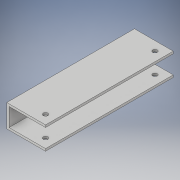
# Autodesk Inventor part: U holder
Saved by Autodesk Inventor 2017 (Build 210142000, 142)
## iProperties
Created: 2019-02-04
Part Number: U holder
Material: Generic
Document SubType Name: Modeling
Designer: S346553810
Density: 1 g/cm^3
Appearance: Default
Author: S346553810
Autodesk Inventor part; units mm, degrees
ref_plane "YZ Plane" through (0, 0, 0) normal (1, 0, 0) x (0, 1, 0)
ref_plane "XZ Plane" through (0, 0, 0) normal (0, 1, 0) x (-1, 0, 0)
ref_plane "XY Plane" through (0, 0, 0) normal (0, 0, 1) x (1, 0, 0)
sketch "Sketch1" plane through (0, 0, 0) normal (0, 0, 1) x (1, 0, 0)
  line L0 (0, 0) -> (-53.975, 0)
  line L1 (-53.975, 0) -> (-53.975, -31.75)
  line L2 (-53.975, -31.75) -> (0, -31.75)
  line L3 (0, -3.175) -> (-50.8, -3.175)
  line L4 (-50.8, -3.175) -> (-50.8, -28.575)
  line L5 (-50.8, -28.575) -> (0, -28.575)
  line L6 (0, -3.175) -> (0, 0)
  line L7 (0, -28.575) -> (0, -31.75)
  dimension "d3" = 3.175
  dimension "d6" = 25.4
  dimension "d7" = 50.8
  constraints: 16 end point, 4 perpendicular, 2 collinear, 1 horizontal, 1 vertical, 2 other
  measures "d3" distance between parallel lines of L0 L3
  measures "d6" distance of L3.end L4.end
  measures "d7" distance of L3.start L3.end
extrude "Extrusion1" add sketch "Sketch1" along normal blind 177.8
sketch "Sketch2" plane through (-53.975, 0, 0) normal (0, 1, 0) x (1, 0, 0)
  circle A0 centre (41.275, -165.1) radius 3.175
  line L0 (53.975, 0) -> (53.975, -177.8) projected
  circle A1 centre (41.275, -12.7) radius 3.175
  line L1 (53.975, -177.8) -> (0, -177.8) projected
  line L2 (53.975, 0) -> (0, 0) projected
  dimension "d8" = 6.35
  dimension "d9" = 12.7
  dimension "d10" = 6.35
  dimension "d11" = 12.7
  dimension "d12" = 12.7
  dimension "d13" = 12.7
  constraints: 2 centre point
  measures "d8" diameter of A0
  measures "d9" distance from line of L0 A0.centre
  measures "d10" diameter of A1
  measures "d11" distance from line of L0 A1.centre
  measures "d12" distance from line of L1 A0.centre
  measures "d13" distance from line of L2 A1.centre
extrude "Extrusion2" cut sketch "Sketch2" against normal through all
body "Solid1"
